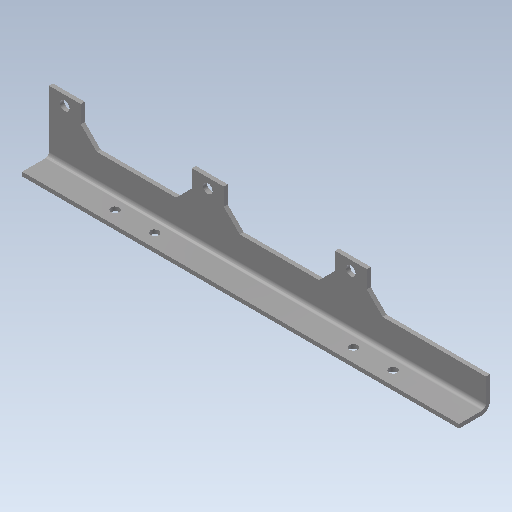
# Autodesk Inventor part: ADSK-MH-10035
Saved by Autodesk Inventor 2020.2 (Build 242310000, 310)
## iProperties
Created: 2008-03-12
Part Number: ADSK-MH-10035
Document SubType Name: Sheet Metal
Designer: R.O'mahony
Density: 7.86 g/cm^3
Mass: 1521.74 g
Surface Area: 857.345 cm^2
Volume: 193.606 cm^3
Material: Steel, Mild
Sheet Metal Rule: Default
Appearance: Steel
Description: Discharge Platform Roller Side Plate
Engineer: Demir Ali
Checked By: Demir Ali
Company: Autodesk Ltd
Author: R.O'mahony
Keywords: Roller Conveyor
Revision Number: A
Autodesk Inventor part; units mm, degrees
ref_plane "YZ Plane" through (0, 0, 0) normal (1, 0, 0) x (0, 1, 0)
ref_plane "XZ Plane" through (0, 0, 0) normal (0, 1, 0) x (-1, 0, 0)
ref_plane "XY Plane" through (0, 0, 0) normal (0, 0, 1) x (1, 0, 0)
sketch "Sketch1" plane through (0, 0, 0) normal (0, 0, 1) x (1, 0, 0)
  circle A0 centre (150, 17) radius 5.25
  circle A1 centre (100, 17) radius 5.25
  line L0 (0, 0) -> (550, 0)
  line L1 (550, 0) -> (550, 70)
  line L2 (550, 70) -> (0, 70)
  circle A2 centre (20, 100) radius 6
  line L3 (40, 70) -> (40, 112)
  line L4 (40, 112) -> (0, 112)
  line L5 (0, 112) -> (0, 0)
  line L6 (0, 34.4774) -> (550, 34.4774) construction
  point P0 (20, 112)
  dimension "d19" = 10.5
  dimension "d20" = 12
  dimension "d21" = 40
  dimension "d22" = 42
  dimension "d23" = 550
  dimension "d25" = 50
  dimension "d26" = 17
  dimension "d27" = 70
  dimension "d28" = 100
  dimension "d29" = 12
  constraints: 14 end point, 4 perpendicular, 4 point on line, 3 centre point, 1 coincident, 1 equal radius, 1 horizontal, 1 horizontal alignment, 1 midpoint, 1 parallel, 1 vertical, 1 vertical alignment
  measures "d19" diameter of A1
  measures "d20" diameter of A2
  measures "d21" distance of L3.end L4.end
  measures "d22" distance of L3.start L3.end
  measures "d23" distance of L0.start L0.end
  measures "d25" distance of A0.centre A1.centre
  measures "d26" distance from line of L0 A1.centre
  measures "d27" distance of L0.end L1.end
  measures "d28" distance from line of L5 A1.centre
  measures "d29" distance from line of L4 A2.centre
extrude "Plate1" add sketch "Sketch1" along normal blind 5 contours A0 | A1 | L5 L2 L1 L0
sheet face with bend "Face2" sketch "Sketch1" thickness 5 toward (0, 0, 1) bend radius 5 relief straight relief width 5 relief depth 2.5 contours L5 L4 L3 L2
bend "Bend2"
extrude "Cut2" cut sketch "Sketch1" along normal blind 5 contours A0 | A1
pattern_linear "Rectangular Pattern1" count 2 spacing 300 along (1, 0, 0) of "Cut2"
fold "Fold1" angle 90 bend radius 5 thickness 5 k factor 0.44 line from (0, 34.4774, 0) to (550, 34.4774, 0) line at bend centre moving side (0, -1, 0) folds toward (0, 0, 1)
pattern_linear "Rectangular Pattern2" count 3 spacing 180 along (1, 0, 0) of "Face2"
chamfer "Corner Chamfer1" distance 20 angle 45 5 edges at (400, 70, 2.5) (360, 70, 2.5) (220, 70, 2.5) (180, 70, 2.5) (40, 70, 2.5)
equation "\"d45\" = Thickness"
equation "\"d56\" = BendReliefWidth"
equation "\"d57\" = BendReliefDepth"
equation "\"d58\" = MinimumRemnant"
equation "\"d59\" = BendRadius"
equation "\"d61\" = BendRadius"
equation "\"d62\" = Thickness"
equation "\"d30\" = BendRadius"
equation "\"d31\" = BendReliefWidth"
equation "\"d33\" = MinimumRemnant"
equation "\"d32\" = BendReliefDepth"
equation "\"d34\" = BendRadius"
equation "\"BendRadius\" = Thickness"
equation "\"BendReliefWidth\" = Thickness"
equation "\"BendReliefDepth\" = 0.5 * Thickness"
equation "\"TransitionRadius\" = BendRadius"
equation "\"JacobiRadiusSize\" = Thickness"
equation "\"d4\" = BendRadius"
equation "\"GapSize\" = Thickness"
equation "\"Thickness\" = 5"
equation "\"MinimumRemnant\" = 10"
body "Solid1"
